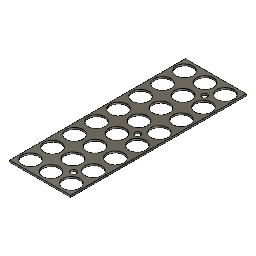
8x3_pcb_mask (Autodesk Fusion 360 design; units mm, degrees)
Autodesk Fusion 360 part; units mm, degrees
sketch "8x3-Edge_Cuts" plane through (0, 0, 0) normal (0, 0, 1) x (1, 0, 0)
  line L0 (83, -29.5) -> (17, -29.5)
  line L1 (17, -29.5) -> (17, -219.1)
  line L2 (83, -219.1) -> (83, -29.5)
  line L3 (17, -219.1) -> (83, -219.1)
sketch "8x3-User_Drawings" plane through (0, 0, 0) normal (0, 0, 1) x (1, 0, 0)
  circle A0 centre (50.0768, -183.65) radius 9
  circle A1 centre (50.0768, -159.95) radius 9
  circle A2 centre (72.0768, -112.55) radius 9
  circle A3 centre (50.0768, -207.35) radius 9
  circle A4 centre (28.0768, -159.95) radius 9
  circle A5 centre (28.0768, -183.65) radius 9
  circle A6 centre (50.0768, -136.25) radius 9
  circle A7 centre (72.0768, -41.45) radius 9
  circle A8 centre (72.0768, -88.85) radius 9
  circle A9 centre (28.0768, -136.25) radius 9
  circle A10 centre (72.0768, -207.35) radius 9
  circle A11 centre (72.0768, -65.15) radius 9
  circle A12 centre (50.0768, -112.55) radius 9
  circle A13 centre (50.0768, -41.45) radius 9
  circle A14 centre (28.0768, -207.35) radius 9
  circle A15 centre (28.0768, -88.85) radius 9
  circle A16 centre (50.0768, -65.15) radius 9
  circle A17 centre (28.0768, -112.55) radius 9
  circle A18 centre (50.0768, -88.85) radius 9
  circle A19 centre (72.0768, -159.95) radius 9
  circle A20 centre (72.0768, -183.65) radius 9
  circle A21 centre (28.0768, -41.45) radius 9
  circle A22 centre (28.0768, -65.15) radius 9
  circle A23 centre (72.0768, -136.25) radius 9
sketch "8x3-User_Comments" plane through (0, 0, 0) normal (0, 0, 1) x (1, 0, 0)
  circle A0 centre (62.08, -53.72) radius 3
  circle A1 centre (62.58, -195.47) radius 3
  circle A2 centre (61.81, -125.54) radius 3
extrude "Extrude1" add sketch "8x3-Edge_Cuts" along normal blind 2
extrude "Extrude2" cut sketch "8x3-User_Comments" sketch "8x3-User_Drawings" along normal blind 2 of sketch 2
